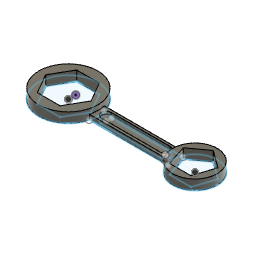
Assignment_02 (Autodesk Fusion 360 design; units mm, degrees)
Autodesk Fusion 360 part; units mm, degrees
note: some values were not read from the file. Set by a fixed rule: which sketch regions a step uses.
sketch "Sketch1" plane through (0, 0, 0) normal (0, 1, 0) x (1, 0, 0)
  line L0 (139.8981, -22.5) -> (146.6336, -1.7705)
  line L1 (146.6336, -1.7705) -> (129, 11.041)
  line L2 (129, 11.041) -> (111.3664, -1.7705)
  line L3 (111.3664, -1.7705) -> (118.1019, -22.5)
  line L4 (118.1019, -22.5) -> (139.8981, -22.5)
  line L5 (11.547, -27.5) -> (23.094, -7.5)
  line L6 (23.094, -7.5) -> (11.547, 12.5)
  line L7 (11.547, 12.5) -> (-11.547, 12.5)
  line L8 (-11.547, 12.5) -> (-23.094, -7.5)
  line L9 (-23.094, -7.5) -> (-11.547, -27.5)
  line L10 (-11.547, -27.5) -> (11.547, -27.5)
  circle A0 centre (0, -7.5) radius 30
  circle A1 centre (129, -7.5) radius 22.5
  line L11 (38.4299, -12.3139) -> (98.4299, -12.3139)
  line L12 (103.4299, -7.3139) -> (103.4299, -7.3123)
  line L13 (98.4299, -2.3142) -> (38.479, -2.3142)
  line L14 (38.7, -2.3142) -> (38.479, -2.3142)
  arc A2 (38.479, -2.3142) -> (38.4299, -12.3139) centre (38.4299, -7.3139) ccw
  arc A3 (103.4299, -7.3123) -> (98.4299, -2.3142) centre (98.4299, -7.3142) ccw
  arc A4 (98.4299, -12.3139) -> (103.4299, -7.3139) centre (98.4299, -7.3139) ccw
  line L15 (28.6408, -15) -> (109.0777, -15)
  line L16 (109.0777, 0) -> (28.6408, 0)
  point P0 (0, -7.5)
  point P1 (129, -7.5)
  point P2 (103.4299, -12.3139)
  dimension "d2" = 20
  dimension "d3" = 60
  dimension "d4" = 45
  dimension "d7" = 5
  constraint coincident P0 A0.centre
  constraint coincident P1 A1.centre
  constraint horizontal L11
  constraint horizontal L13
  constraint tangent L11 A2
  constraint tangent L13 A3
  constraint equal A2 A3
  constraint coincident P2 L11
  constraint coincident P2 L12
  constraint tangent L11 A4
  constraint tangent L12 A4
  constraint equal A2 A4
  constraint horizontal L14
  constraint horizontal L15
  constraint horizontal L16
  measures "d2" distance of P0 L10
  measures "d3" diameter of A0
  measures "d4" diameter of A1
  measures "d7" radius of A2
extrude "Extrude1" add sketch "Sketch1" along normal blind 10 contours A0 | A1 makes body 1 at (-13.6863, 6.6667, 34.1962) makes body 2 at (151.3882, 3.3333, 9.7403)
extrude "Extrude2" add sketch "Sketch1" along normal blind 5 contours A0 A1 L15 L16 bodies 1 2
extrude "Extrude3" add sketch "Sketch1" along normal blind 2.5 contours L11 L13 L14 A2 A3 A4 bodies 1
